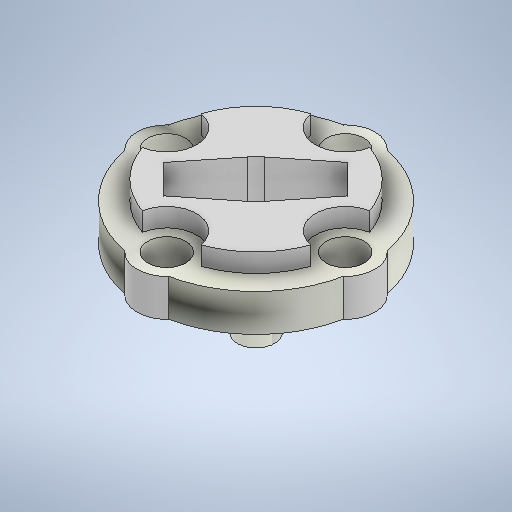
# Autodesk Inventor part: Redesign_Spinner
Saved by Autodesk Inventor 2025.1 (Build 291241000, 241)
## iProperties
Created: 2024-12-23
Part Number: Redesign_Spinner
Material: Generic
Document SubType Name: Modeling
Designer: m_kni
Density: 1 g/cm^3
Appearance: Default
Finish1_Area: 1468.638 mm^2
Finish1_Appearance: Running - Light Gray
Finish1_Process: Prime/Paint RAL 3018
Finish1_Description: Prime/Paint RAL 3018
Finish1_ShortDescription: RAL 3018
Finish1_Thickness: 0.050 mm
Author: m_kni
## iProperties of the stored document Redesign_Spinner_3DPrint.ipt
Created: 2025-01-30
Part Number: Redesign_Spinner_3DPrint
Material: Generic
Document SubType Name: Modeling
Designer: m_kni
Density: 1 g/cm^3
Appearance: Default
Author: m_kni
Autodesk Inventor part; units mm, degrees
ref_plane "YZ Plane" through (0, 0, 0) normal (1, 0, 0) x (0, 1, 0)
ref_plane "XZ Plane" through (0, 0, 0) normal (0, 1, 0) x (-1, 0, 0)
ref_plane "XY Plane" through (0, 0, 0) normal (0, 0, 1) x (1, 0, 0)
sketch "Sketch1" plane through (0, 0, 0) normal (0, 1, 0) x (-1, 0, 0)
  circle A0 centre (0, 0) radius 2.495
  dimension "d0" = 4.99
  constraints: 1 centre point, 1 coincident
  measures "d0" diameter of A0
extrude "Extrusion1" add sketch "Sketch1" along normal blind 10.4
sketch "Sketch2" plane through (0, 10.4, 0) normal (0, 1, 0) x (1, 0, 0)
  circle A0 centre (0, 0) radius 12
  circle A1 centre (-12, 0) radius 1.5
  circle A2 centre (-12, 0) radius 2.55
  circle A3 centre (0, -12) radius 1.5
  circle A4 centre (0, -12) radius 2.55
  circle A5 centre (12, 0) radius 1.5
  circle A6 centre (12, 0) radius 2.55
  circle A7 centre (0, 12) radius 1.5
  circle A8 centre (0, 12) radius 2.55
  circle A9 centre (0, 0) radius 14.9832
  circle A10 centre (12, 0) radius 4
  circle A11 centre (0, -12) radius 4
  circle A12 centre (-12, 0) radius 4
  circle A13 centre (0, 12) radius 4
  point P0 (2.9628, -14.6873)
  point P1 (-2.9628, -14.6873)
  point P2 (-14.6873, -2.9628)
  point P3 (-14.6873, 2.9628)
  point P4 (-2.9628, 14.6873)
  point P5 (2.9628, 14.6873)
  point P6 (14.6873, 2.9628)
  point P7 (14.6873, -2.9628)
  dimension "d3" = 24
  dimension "d4" = 3
  dimension "d5" = 5.1
  dimension "d8" = 360
  dimension "d22" = 8
  dimension "d23" = 8
  dimension "d24" = 8
  dimension "d25" = 8
  constraints: 14 centre point, 6 coincident, 2 point on circle, 17 other
  measures "d3" diameter of A0
  measures "d4" diameter of A1
  measures "d5" diameter of A2
  measures "d22" diameter of A10
  measures "d23" diameter of A11
  measures "d24" diameter of A12
  measures "d25" diameter of A13
extrude "Extrusion2" add sketch "Sketch2" along normal blind 5 contours A6 A0 A10 | A0 A10 A9 A6 | A10 A0 A11 A12 A13 | A0 A13 A9 A10 | A10 A9 A11 A0 | A13 A0 A8 | A0 A8 A13 A9 | A10 A9 | A11 A9 A0 A4 | A0 A4 A11 | A0 A12 A9 A13 | A9 A13 | A11 A9 A12 A0 | A11 A9 | A12 A0 A2 | A0 A2 A12 A9 | A9 A12
sketch "Sketch3" plane through (0, 15.4, 0) normal (0, 1, 0) x (1, 0, 0)
  circle A0 centre (0, 0) radius 2.495 projected
  circle A1 centre (0, 0) radius 1.05
  dimension "d13" = 2.1
  constraints: 1 centre point, 1 coincident
  measures "d13" diameter of A1
extrude "Extrusion3" cut sketch "Sketch3" against normal blind 18.3375 contours A1
sketch "Sketch5" plane through (0, 0, 0) normal (0, -1, 0) x (1, 0, 0)
  circle A0 centre (0, 0) radius 1.05 projected
  circle A1 centre (0, 0) radius 1.825
  dimension "d19" = 3.65
  constraints: 1 centre point, 1 coincident
  measures "d19" diameter of A1
extrude "Extrusion5" cut sketch "Sketch5" against normal blind 12.4
sketch "Sketch6" plane through (0, 15.4, 0) normal (0, 1, 0) x (1, 0, 0)
  circle A0 centre (0, 0) radius 2
  circle A1 centre (0, 0) radius 1.05
  circle A2 centre (0, 0) radius 2.4
  circle A3 centre (0, 0) radius 1.05 projected
  circle A4 centre (0, 0) radius 3
  dimension "d26" = 4
  dimension "d30" = 4.8
  dimension "d31" = 6
  constraints: 4 centre point, 4 coincident
  measures "d26" diameter of A0
  measures "d30" diameter of A2
  measures "d31" diameter of A4
extrude "Extrusion6" add sketch "Sketch6" along normal blind 2.5 contours A4
sketch "Sketch8" plane through (0, 15.4, 0) normal (0, 1, 0) x (1, 0, 0)
  circle A0 centre (0, -12) radius 2.55 projected
  circle A1 centre (-12, 0) radius 2.55 projected
  circle A2 centre (0, 12) radius 2.55 projected
  circle A3 centre (12, 0) radius 2.55 projected
  circle A4 centre (0, 0) radius 12
  circle A5 centre (0, -12) radius 4
  circle A6 centre (-12, 0) radius 4
  circle A7 centre (0, 12) radius 4
  circle A8 centre (12, 0) radius 4
  circle A9 centre (0, 0) radius 3
  point P0 (11.3333, -3.9441)
  point P1 (11.3333, 3.9441)
  point P2 (3.9441, 11.3333)
  point P3 (-3.9441, 11.3333)
  point P4 (-11.3333, 3.9441)
  point P5 (-11.3333, -3.9441)
  point P6 (-3.9441, -11.3333)
  point P7 (3.9441, -11.3333)
  constraints: 6 coincident, 5 centre point, 3 other
extrude "Extrusion8" add sketch "Sketch8" along normal up to surface (2.5 mm away) contours A5 A4 A6 A7 A8
sketch "Sketch9" plane through (0, 17.9, 0) normal (0, 1, 0) x (1, 0, 0)
  arc A0 (-11.3333, -3.9441) -> (-3.9441, -11.3333) centre (0, 0) ccw projected
  line L0 (0, 0) -> (-6.1872, -6.1872)
  line L1 (0, 0) -> (8.75, 0) construction
  circle A1 centre (0, 0) radius 3.75
  circle A2 centre (0, 0) radius 1.05 projected
  line L2 (2.6517, -2.6517) -> (12.6517, -2.6517) construction
  line L3 (-2.6517, 2.6517) -> (7.3483, 2.6517) construction
  circle A3 centre (0, 0) radius 2.4
  line L4 (-6.1872, -6.1872) -> (-8.1317, -4.2426)
  line L5 (-6.1872, -6.1872) -> (-4.2426, -8.1317)
  line L6 (-4.2426, -8.1317) -> (2.6517, -2.6517)
  line L7 (-8.1317, -4.2426) -> (-2.6517, 2.6517)
  line L8 (-2.6517, 2.6517) -> (2.6517, -2.6517)
  line L9 (6.1872, 6.1872) -> (4.2426, 8.1317)
  line L10 (6.1872, 6.1872) -> (8.1317, 4.2426)
  line L11 (8.1317, 4.2426) -> (2.6517, -2.6517)
  line L12 (4.2426, 8.1317) -> (-2.6517, 2.6517)
  point P0 (3.1816, -1.985)
  point P1 (-1.985, 3.1816)
  point P2 (-3.1816, 1.985)
  point P3 (1.985, -3.1816)
  dimension "d45" = 8.75
  dimension "d46" = 135
  dimension "d47" = 7.5
  dimension "d64" = 2.75
  dimension "d65" = 2.75
  constraints: 26 end point, 3 horizontal, 3 symmetric about line, 2 centre point, 2 coincident, 2 point on circle, 1 equal length
  measures "d45" distance of L0.start L0.end
  measures "d46" angle of L0 L1
  measures "d47" diameter of A1
  measures "d64" distance of L0.end L4.end
  measures "d65" distance of L0.end L5.end
extrude "Extrusion9" cut sketch "Sketch9" against normal blind 6
sketch "Sketch10" plane through (0, 0, 0) normal (0, -1, 0) x (1, 0, 0)
  circle A0 centre (0, 0) radius 1.825 projected
  circle A1 centre (0, 0) radius 1.825
  constraints: 1 centre point, 1 coincident, 1 concentric
extrude "Extrusion10" add sketch "Sketch10" against normal up to surface (15.4 mm away)
sketch "Sketch11" plane through (0, 10.4, 0) normal (0, -1, 0) x (1, 0, 0)
  circle A0 centre (0, 0) radius 3.25
  dimension "d56" = 6.5
  constraints: 1 centre point, 1 coincident
  measures "d56" diameter of A0
extrude "Extrusion11" add sketch "Sketch11" along normal blind 5.4
fillet "Fillet5" radius 5.175 1 edges at (-3.25, 10.4, 0)
sketch "Sketch12" plane through (0, 15.4, 0) normal (0, 1, 0) x (1, 0, 0)
  circle A0 centre (0, 0) radius 2.4 projected
extrude "Extrusion12" cut sketch "Sketch12" against normal up to surface (3.5 mm away)
body "Solid1"
